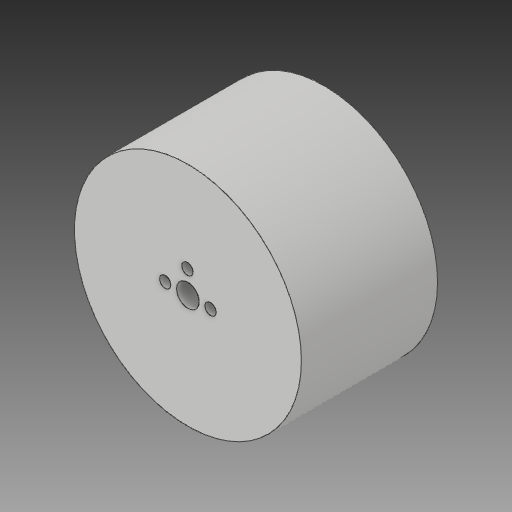
# Autodesk Inventor part: ローラー
Saved by Autodesk Inventor 2019 (Build 230136000, 136)
## iProperties
Created: 2020-09-22
Part Number: ローラー
Material: 一般
Document SubType Name: Modeling
Designer: Toshihito
Density: 1 g/cm^3
Appearance: 既定
Mass: 462.992 g
Surface Area: 389.95 cm^2
Volume: 462.992 cm^3
Author: Toshihito
Autodesk Inventor part; units mm, degrees
ref_plane "YZ Plane" through (0, 0, 0) normal (1, 0, 0) x (0, 1, 0)
ref_plane "XZ Plane" through (0, 0, 0) normal (0, 1, 0) x (-1, 0, 0)
ref_plane "XY Plane" through (0, 0, 0) normal (0, 0, 1) x (1, 0, 0)
sketch "スケッチ1" plane through (0, 0, 0) normal (0, 0, 1) x (1, 0, 0)
  circle A0 centre (0, 0) radius 50
  dimension "d0" = 100
  constraints: 1 centre point, 1 coincident
  measures "d0" diameter of A0
extrude "押し出し1" add sketch "スケッチ1" along normal blind 60
sketch "スケッチ2" plane through (0, 0, 60) normal (0, 0, 1) x (1, 0, 0)
  point P0 (0, 0)
  point P1 (0, 0)
  constraints: 1 coincident
hole "穴1" at (0, 0, 60) direction (0, 0, -1) diameter 10 depth 60 tip angle 118
sketch "スケッチ3" plane through (0, 0, 60) normal (0, 0, 1) x (1, 0, 0)
  circle A0 centre (0, 0) radius 5 projected
  circle A1 centre (0, 0) radius 10 construction
  point P0 (-9.9993, 0.1214)
  point P1 (-0.1795, 9.9984)
  point P2 (9.997, -0.246)
  dimension "d17" = 20
  constraints: 3 point on circle, 1 centre point, 1 coincident
  measures "d17" diameter of A1
hole "穴2" at (-9.9993, 0.1214, 60) at (-0.1795, 9.9984, 60) at (9.997, -0.246, 60) direction (0, 0, -1) diameter 5 depth 60 tip angle 118
